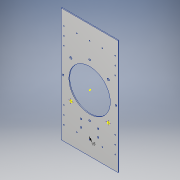
# Autodesk Inventor part: ベアリング板
Saved by Autodesk Inventor 2019 (Build 230136000, 136)
## iProperties
Created: 2020-10-01
Part Number: ベアリング板
Material: アルミニウム 6061
Document SubType Name: Modeling
Designer: Toshihito
Density: 2.7 g/cm^3
Appearance: アルミニウム - フラット
Author: Toshihito
Autodesk Inventor part; units mm, degrees
ref_plane "YZ Plane" through (0, 0, 0) normal (1, 0, 0) x (0, 1, 0)
ref_plane "XZ Plane" through (0, 0, 0) normal (0, 1, 0) x (-1, 0, 0)
ref_plane "XY Plane" through (0, 0, 0) normal (0, 0, 1) x (1, 0, 0)
sketch "スケッチ1" plane through (0, 0, 0) normal (0, 0, 1) x (1, 0, 0)
  line L0 (-100, 100) -> (100, 100)
  line L1 (100, 100) -> (100, -100)
  line L2 (100, -100) -> (-100, -100)
  line L3 (-100, -100) -> (-100, 100)
  line L4 (-100, 100) -> (100, -100) construction
  line L5 (100, 100) -> (-100, -100) construction
  circle A0 centre (0, 0) radius 92.5 construction
  circle A1 centre (-65.4074, 65.4074) radius 4
  circle A2 centre (65.4074, 65.4074) radius 4
  circle A3 centre (65.4074, -65.4074) radius 4
  circle A4 centre (-65.4074, -65.4074) radius 4
  dimension "d0" = 200
  dimension "d1" = 200
  dimension "d2" = 185
  dimension "d3" = 8
  dimension "d4" = 8
  dimension "d5" = 8
  dimension "d6" = 8
  constraints: 12 end point, 5 centre point, 4 point on circle, 4 point on line, 2 midpoint, 2 parallel, 1 coincident, 1 horizontal, 1 perpendicular
  measures "d0" distance of L1.end L2.end
  measures "d1" distance of L0.end L1.end
  measures "d2" diameter of A0
  measures "d3" diameter of A1
  measures "d4" diameter of A2
  measures "d5" diameter of A3
  measures "d6" diameter of A4
extrude "押し出し1" add sketch "スケッチ1" along normal blind 3
sketch "スケッチ2" plane through (0, 0, 0) normal (0, 0, -1) x (-1, 0, 0)
  circle A0 centre (0, 0) radius 72.5
  dimension "d9" = 145
  constraints: 1 centre point, 1 coincident
  measures "d9" diameter of A0
extrude "押し出し2" cut sketch "スケッチ2" against normal blind 10
sketch "スケッチ3" plane through (0, 0, 3) normal (0, 0, 1) x (1, 0, 0)
  circle A0 centre (-65.4074, -65.4074) radius 4 projected
  circle A1 centre (65.4074, -65.4074) radius 4 projected
  point P0 (0, 0)
  constraints: 2 coincident
sketch "スケッチ4" plane through (-100, -100, 0) normal (0, -1, 0) x (1, 0, 0)
  line L0 (0, 0) -> (0, 3) projected
  line L1 (200, 0) -> (200, 3) projected
  line L2 (0, 3) -> (200, 3)
  line L3 (200, 3) -> (200, 0)
  line L4 (200, 0) -> (0, 0)
  line L5 (0, 0) -> (0, 3)
  point P0 (100, 0)
  constraints: 8 end point, 2 parallel, 1 horizontal, 1 perpendicular
extrude "押し出し3" add sketch "スケッチ4" along normal blind 100
sketch "スケッチ7" plane through (0, 0, 0) normal (0, 0, -1) x (-1, 0, 0)
  circle A0 centre (30, -128) radius 3
  circle A1 centre (-30, -128) radius 3
  circle A2 centre (30, -102) radius 3
  circle A3 centre (-30, -102) radius 3
  point P0 (0, -115)
  dimension "d40" = 6
  dimension "d41" = 6
  dimension "d42" = 6
  dimension "d43" = 6
  constraints: 4 centre point
  measures "d40" diameter of A0
  measures "d41" diameter of A1
  measures "d42" diameter of A2
  measures "d43" diameter of A3
sketch "スケッチ8" plane through (-100, 100, 0) normal (0, 1, 0) x (1, 0, 0)
  line L0 (0, 0) -> (200, 0) projected
  line L1 (200, 0) -> (200, -3) projected
  line L2 (0, 0) -> (200, 0)
  line L3 (200, 0) -> (200, -3)
  line L4 (200, -3) -> (0, -3)
  line L5 (0, -3) -> (0, 0)
  point P0 (100, 0)
  constraints: 8 end point, 2 parallel, 1 horizontal, 1 perpendicular
extrude "押し出し7" add sketch "スケッチ8" along normal blind 100
sketch "スケッチ9" plane through (0, 0, 0) normal (0, 0, -1) x (-1, 0, 0)
  circle A0 centre (0, -120) radius 30
  circle A1 centre (0, 0) radius 102.5
  circle A2 centre (0, -150) radius 1.65
  circle A3 centre (-45, -150) radius 1.65
  circle A4 centre (-90, -150) radius 1.65
  circle A5 centre (45, -150) radius 1.65
  circle A6 centre (90, -150) radius 1.65
  circle A7 centre (-90, 150) radius 1.65
  circle A8 centre (-45, 150) radius 1.65
  circle A9 centre (0, 150) radius 1.65
  circle A10 centre (45, 150) radius 1.65
  circle A11 centre (90, 150) radius 1.65
  dimension "d44" = 60
  dimension "d47" = 205
  dimension "d60" = 3.3
  dimension "d61" = 3.3
  dimension "d62" = 3.3
  dimension "d63" = 3.3
  dimension "d64" = 3.3
  dimension "d65" = 3.3
  dimension "d66" = 3.3
  dimension "d67" = 3.3
  dimension "d68" = 3.3
  dimension "d69" = 3.3
  constraints: 11 centre point, 3 coincident, 1 vertical alignment, 2 other
  measures "d47" diameter of A1
  measures "d60" diameter of A2
  measures "d61" diameter of A3
  measures "d62" diameter of A4
  measures "d63" diameter of A5
  measures "d64" diameter of A6
  measures "d65" diameter of A7
  measures "d66" diameter of A8
  measures "d67" diameter of A9
  measures "d68" diameter of A10
  measures "d69" diameter of A11
extrude "押し出し8" cut sketch "スケッチ7" against normal blind 10
sketch "スケッチ10" plane through (0, 0, 0) normal (0, 0, -1) x (-1, 0, 0)
  point P0 (0, 0)
sketch "スケッチ11" plane through (0, 0, 0) normal (0, 0, -1) x (-1, 0, 0)
  point P0 (0, 0)
extrude "押し出し10" cut sketch "スケッチ9" against normal blind 10 contours A2 A0 | A0 A2 | A3 | A4 | A5 | A6 | A7 | A8 | A9 | A10 | A11
sketch "スケッチ12" plane through (0, 0, 0) normal (0, 0, -1) x (-1, 0, 0)
  circle A0 centre (0, -150) radius 1.65 projected
  circle A1 centre (0, -150) radius 7.5
  point P0 (0, 0)
  dimension "d72" = 15
  constraints: 1 centre point, 1 coincident
  measures "d72" diameter of A1
sketch "スケッチ13" plane through (0, 0, 0) normal (0, 0, -1) x (-1, 0, 0)
  circle A0 centre (-90, -90) radius 1.65
  circle A1 centre (90, -90) radius 1.65
  circle A2 centre (-90, 90) radius 1.65
  circle A3 centre (90, 90) radius 1.65
  circle A4 centre (-90, -120) radius 1.65
  circle A5 centre (90, -120) radius 1.65
  circle A6 centre (-90, 120) radius 1.65
  circle A7 centre (90, 120) radius 1.65
  point P0 (0, 0)
  dimension "d81" = 3.3
  dimension "d82" = 3.3
  dimension "d83" = 3.3
  dimension "d84" = 3.3
  dimension "d85" = 3.3
  dimension "d86" = 3.3
  dimension "d87" = 3.3
  dimension "d88" = 3.3
  constraints: 8 centre point
  measures "d81" diameter of A0
  measures "d82" diameter of A1
  measures "d83" diameter of A2
  measures "d84" diameter of A3
  measures "d85" diameter of A4
  measures "d86" diameter of A5
  measures "d87" diameter of A6
  measures "d88" diameter of A7
sketch "スケッチ14" plane through (0, 0, 0) normal (0, 0, -1) x (-1, 0, 0)
  circle A0 centre (0, 0) radius 92.5
  circle A1 centre (0, -92.5) radius 3
  circle A2 centre (-92.5, 0) radius 3
  circle A3 centre (0, 92.5) radius 3
  circle A4 centre (92.5, 0) radius 3
  dimension "d74" = 185
  dimension "d75" = 6
  dimension "d76" = 6
  dimension "d77" = 6
  dimension "d78" = 6
  constraints: 5 centre point, 4 point on circle, 1 coincident
  measures "d74" diameter of A0
  measures "d75" diameter of A1
  measures "d76" diameter of A2
  measures "d77" diameter of A3
  measures "d78" diameter of A4
extrude "押し出し11" cut sketch "スケッチ14" against normal blind 10 contours A0 A4 | A0 A4 | A3 A0 | A0 A3 | A1 A0 | A0 A1 | A2 A0 | A0 A2
extrude "押し出し12" cut sketch "スケッチ13" against normal blind 10
